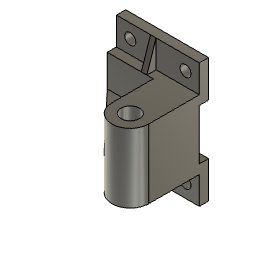
A2_AI22BTECH11005_4 (Autodesk Fusion 360 design; units mm, degrees)
Autodesk Fusion 360 part; units mm, degrees
note: some values were not read from the file. Set by a fixed rule: which sketch regions a step uses.
sketch "Sketch1" plane through (0, 0, 0) normal (0, 0, 1) x (1, 0, 0)
  line L0 (-50, 20) -> (40, 20)
  line L1 (40, 20) -> (40, 0)
  line L2 (40, 0) -> (40, -35)
  line L3 (0, -35) -> (0, 10)
  line L4 (0, 10) -> (-50, 10)
  line L5 (-50, 10) -> (-50, 20)
  arc A0 (0, -35) -> (40, -35) centre (20, -35) ccw
  arc A1 (10, -35) -> (30, -35) centre (20, -35) ccw
  arc A2 (30, -35) -> (10, -35) centre (20, -35) ccw
  line L6 (-50, 20) -> (-50, 30)
  line L7 (-50, 30) -> (40, 30)
  line L8 (40, 30) -> (40, 20)
  constraint horizontal L0
  constraint perpendicular L0 L1
  constraint perpendicular L0 L2
  constraint perpendicular L0 L3
  constraint perpendicular L3 L4
  constraint perpendicular L0 L5
  constraint concentric A0 A1
  constraint concentric A1 A2
  constraint perpendicular L0 L6
  constraint perpendicular L6 L7
  constraint perpendicular L0 L8
extrude "Extrude1" add sketch "Sketch1" along normal blind 34.5 contours L0 L1 L2 L3 L4 L5 A0
extrude "Extrude3" add sketch "Sketch1" along normal blind 10 and the other way blind 30 contours L0 L6 L7 L8
ref_plane "WorkPlane1" through (-5, -17.5, 34.5) normal (0, 0, 1) x (1, 0, 0)
sketch "Sketch2" plane through (-5, -17.5, 34.5) normal (0, 0, 1) x (1, 0, 0)
  line L0 (-45, 37.5) -> (-45, 27.5)
  line L1 (-45, 27.5) -> (5, 27.5)
  arc A0 (5, -17.5) -> (5.1544, -19.9807) centre (25, -17.5) ccw
  arc A1 (5.1544, -19.9807) -> (10.4585, -31.2312) centre (25, -17.5) ccw
  line L2 (-45, 27.5) -> (10.4585, -31.2312)
  line L3 (5, 27.5) -> (5, -17.5)
  constraint vertical L0
  constraint perpendicular L0 L1
  constraint concentric A0 A1
  constraint tangent A1 L2
  constraint perpendicular L1 L3
extrude "Extrude4" add sketch "Sketch2" 1 faces at (20.2491, 1.6573, 34.5) along normal blind 3
sketch "Sketch4" plane through (0, 20, 0) normal (0, -1, 0) x (1, 0, 0)
  line L0 (40, 0) -> (-50, 0)
  line L1 (-50, 0) -> (-50, -30)
  line L2 (-50, -30) -> (40, -30)
  line L3 (40, -30) -> (40, 0)
  line L4 (-50, 0) -> (-50, -15)
  line L5 (-50, -15) -> (-30, -15)
  line L6 (-30, -15) -> (20, -15)
  line L7 (20, -15) -> (40, -15)
  circle A0 centre (-35, -15) radius 6
  circle A1 centre (25, -15) radius 6
  dimension "d17" = 12
  dimension "d18" = 12
  constraint coincident L0.end L1.start
  constraint midpoint L1 L4.end
  constraint perpendicular L3 L5
  constraint perpendicular L3 L6
  constraint midpoint L3 L7.end
  constraint perpendicular L3 L7
  constraint coincident L5 A0.centre
  constraint coincident L7 A1.centre
  measures "d17" diameter of A0
  measures "d18" diameter of A1
extrude "Extrude7" cut sketch "Sketch4" against normal blind 10 contours L6 L7 A1 | L6 L7 A1 | L5 L6 A0 | L5 L6 A0
ref_plane "WorkPlane3" through (-13, 20, 3.75) normal (-1, 0, 0) x (0, -1, 0)
sketch "Sketch5" plane through (-13, 20, 3.75) normal (-1, 0, 0) x (0, 1, 0)
  line L0 (-10, 3.75) -> (0, 3.75)
  line L1 (0, 3.75) -> (0, 33.75)
  line L2 (0, 33.75) -> (-10, 3.75)
  constraint horizontal L0
  constraint perpendicular L0 L1
extrude "Extrude8" add sketch "Sketch5" against normal blind 6
mirror "Mirror1" about plane through (-5, -17.5, 37.5) normal (0, 0, 1) of bodies 1 merged
